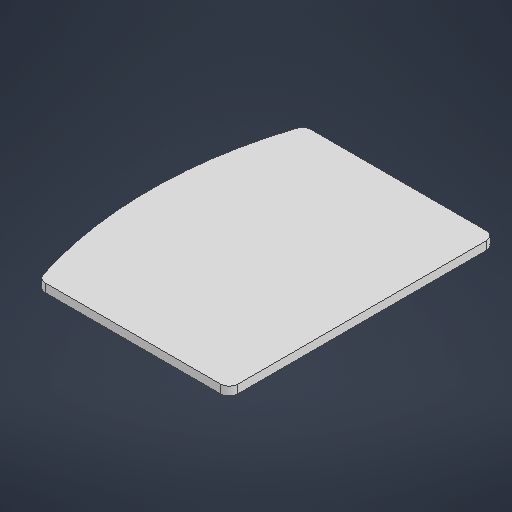
# Autodesk Inventor part: Motorplatine
Saved by Autodesk Inventor 2025.3 (Build 293356000, 356)
## iProperties
Created: 2025-05-31
Part Number: Motorplatine
Material: Generisch
Document SubType Name: Modeling
Designer: theod
Density: 1 g/cm^3
Appearance: Vorgabe
Author: theod
Autodesk Inventor part; units mm, degrees
ref_plane "YZ Plane" through (0, 0, 0) normal (1, 0, 0) x (0, 1, 0)
ref_plane "XZ Plane" through (0, 0, 0) normal (0, 1, 0) x (-1, 0, 0)
ref_plane "XY Plane" through (0, 0, 0) normal (0, 0, 1) x (1, 0, 0)
sketch "Skizze1" plane through (0, 0, 0) normal (0, 0, 1) x (1, 0, 0)
  circle A0 centre (-39, 91.781) radius 1.6
  circle A1 centre (39, 91.781) radius 1.6
  circle A2 centre (-44.3776, -92.6293) radius 1.6
  circle A3 centre (92.6293, 44.3776) radius 1.6
  circle A4 centre (-92.6293, -44.3776) radius 1.6
  circle A5 centre (44.3776, -92.6293) radius 1.6
  circle A6 centre (92.6293, -44.3776) radius 1.6
  circle A7 centre (-92.6293, 44.3776) radius 1.6
  arc A8 (-95.4893, -49.3765) -> (-92.2985, -49.8721) centre (-93.7128, -48.4579) ccw
  line L0 (-90.1561, -47.7297) -> (-92.2985, -49.8721)
  arc A9 (-76.014, -47.7297) -> (-90.1561, -47.7297) centre (-83.085, -54.8008) ccw
  line L1 (-47.7297, -76.014) -> (-76.014, -47.7297)
  arc A10 (-47.7297, -90.1561) -> (-47.7297, -76.014) centre (-54.8008, -83.085) ccw
  line L2 (-49.8721, -92.2985) -> (-47.7297, -90.1561)
  arc A11 (-49.8721, -92.2985) -> (-49.3766, -95.4893) centre (-48.4579, -93.7128) ccw
  arc A12 (-49.3766, -95.4893) -> (49.3765, -95.4893) centre (0, 0) ccw
  arc A13 (49.3765, -95.4893) -> (49.8721, -92.2985) centre (48.4579, -93.7128) ccw
  line L3 (47.7297, -90.1561) -> (49.8721, -92.2985)
  arc A14 (47.7297, -76.014) -> (47.7297, -90.1561) centre (54.8008, -83.085) ccw
  line L4 (76.014, -47.7297) -> (47.7297, -76.014)
  arc A15 (90.1561, -47.7297) -> (76.014, -47.7297) centre (83.085, -54.8008) ccw
  line L5 (92.2985, -49.8721) -> (90.1561, -47.7297)
  arc A16 (92.2985, -49.8721) -> (95.4893, -49.3766) centre (93.7128, -48.4579) ccw
  arc A17 (95.4893, -49.3766) -> (95.4893, 49.3765) centre (0, 0) ccw
  arc A18 (95.4893, 49.3765) -> (92.2985, 49.8721) centre (93.7128, 48.4579) ccw
  line L6 (90.1561, 47.7297) -> (92.2985, 49.8721)
  arc A19 (76.014, 47.7297) -> (90.1561, 47.7297) centre (83.085, 54.8008) ccw
  line L7 (47.7297, 76.014) -> (76.014, 47.7297)
  arc A20 (47.7297, 90.1561) -> (47.7297, 76.014) centre (54.8008, 83.085) ccw
  line L8 (49.8721, 92.2985) -> (47.7297, 90.1561)
  arc A21 (49.8721, 92.2985) -> (49.3766, 95.4893) centre (48.4579, 93.7128) ccw
  arc A22 (49.3766, 95.4893) -> (38.3499, 100.4268) centre (0, 0) ccw
  arc A23 (38.3499, 100.4268) -> (35.7063, 99.0826) centre (37.6364, 98.5584) ccw
  arc A24 (28.7451, 85.4847) -> (35.7063, 99.0826) centre (0, 108.781) ccw
  arc A25 (20.9762, 81.781) -> (28.7451, 85.4847) centre (20.9762, 91.781) ccw
  line L9 (20.9762, 81.781) -> (-20.9762, 81.781)
  arc A26 (-28.7451, 85.4847) -> (-20.9762, 81.781) centre (-20.9762, 91.781) ccw
  arc A27 (-35.7063, 99.0826) -> (-28.7451, 85.4847) centre (0, 108.781) ccw
  arc A28 (-35.7063, 99.0826) -> (-38.3499, 100.4268) centre (-37.6364, 98.5584) ccw
  arc A29 (-38.3499, 100.4268) -> (-49.3765, 95.4893) centre (0, 0) ccw
  arc A30 (-49.3765, 95.4893) -> (-49.8721, 92.2985) centre (-48.4579, 93.7128) ccw
  line L10 (-47.7297, 90.1561) -> (-49.8721, 92.2985)
  arc A31 (-47.7297, 76.014) -> (-47.7297, 90.1561) centre (-54.8008, 83.085) ccw
  line L11 (-76.014, 47.7297) -> (-47.7297, 76.014)
  arc A32 (-90.1561, 47.7297) -> (-76.014, 47.7297) centre (-83.085, 54.8008) ccw
  line L12 (-92.2985, 49.8721) -> (-90.1561, 47.7297)
  arc A33 (-92.2985, 49.8721) -> (-95.4893, 49.3766) centre (-93.7128, 48.4579) ccw
  arc A34 (-95.4893, 49.3766) -> (-95.4893, -49.3765) centre (0, 0) ccw
  circle A35 centre (-67.8822, 48.7904) radius 1.6
  circle A36 centre (-48.7904, 67.8822) radius 1.6
  circle A37 centre (-67.8822, -48.7904) radius 1.6
  circle A38 centre (-48.7904, -67.8823) radius 1.6
  circle A39 centre (48.7904, -67.8823) radius 1.6
  circle A40 centre (67.8823, -48.7904) radius 1.6
  circle A41 centre (67.8823, 48.7904) radius 1.6
  circle A42 centre (48.7904, 67.8822) radius 1.6
  line L13 (48.7904, 67.8822) -> (67.8823, 48.7904) construction
  line L14 (70.7107, 45.9619) -> (45.9619, 70.7107) construction
  line L15 (67.1751, 42.4264) -> (42.4264, 67.1751)
  line L16 (42.4264, 67.1751) -> (49.4975, 74.2462)
  line L17 (49.4975, 74.2462) -> (74.2462, 49.4975)
  line L18 (74.2462, 49.4975) -> (67.1751, 42.4264)
  line L19 (67.1751, 42.4264) -> (49.4975, 74.2462) construction
  line L20 (42.4264, 67.1751) -> (74.2462, 49.4975) construction
  line L21 (0, 0) -> (61.8718, 61.8718) construction
  line L22 (61.8718, 61.8718) -> (13.7886, 13.7886) construction
  line L23 (67.5287, 56.215) -> (19.4454, 8.1317)
  line L24 (19.4454, 8.1317) -> (8.1317, 19.4454)
  line L25 (8.1317, 19.4454) -> (56.215, 67.5287)
  line L26 (56.215, 67.5287) -> (67.5287, 56.215)
  line L27 (67.5287, 56.215) -> (8.1317, 19.4454) construction
  line L28 (19.4454, 8.1317) -> (56.215, 67.5287) construction
  line L29 (-74.2462, 49.4975) -> (-49.4975, 74.2462)
  line L30 (-49.4975, 74.2462) -> (-42.4264, 67.1751)
  line L31 (-56.215, 67.5287) -> (-8.1317, 19.4454)
  line L32 (-42.4264, 67.1751) -> (-67.1751, 42.4264)
  line L33 (-19.4454, 8.1317) -> (-67.5287, 56.215)
  line L34 (-67.1751, 42.4264) -> (-74.2462, 49.4975)
  line L35 (-8.1317, 19.4454) -> (-19.4454, 8.1317)
  line L36 (-49.4975, -74.2462) -> (-74.2462, -49.4975)
  line L37 (-74.2462, -49.4975) -> (-67.1751, -42.4264)
  line L38 (-67.5287, -56.215) -> (-19.4454, -8.1317)
  line L39 (-67.1751, -42.4264) -> (-42.4264, -67.1751)
  line L40 (-8.1317, -19.4454) -> (-56.215, -67.5287)
  line L41 (-42.4264, -67.1751) -> (-49.4975, -74.2462)
  line L42 (-19.4454, -8.1317) -> (-8.1317, -19.4454)
  line L43 (74.2462, -49.4975) -> (49.4975, -74.2462)
  line L44 (49.4975, -74.2462) -> (42.4264, -67.1751)
  line L45 (56.215, -67.5287) -> (8.1317, -19.4454)
  line L46 (42.4264, -67.1751) -> (67.1751, -42.4264)
  line L47 (19.4454, -8.1317) -> (67.5287, -56.215)
  line L48 (67.1751, -42.4264) -> (74.2462, -49.4975)
  line L49 (8.1317, -19.4454) -> (19.4454, -8.1317)
  circle A43 centre (-14.902, -0.6571) radius 1.4
  circle A44 centre (14.732, 5.2251) radius 1.4
  circle A45 centre (0, 0) radius 4.85
  circle A46 centre (-22.9365, 16.8843) radius 1.6
  circle A47 centre (-22.9365, 16.8843) radius 1.6
  circle A48 centre (22.7665, 22.7665) radius 1.6
  circle A49 centre (22.7665, 22.7665) radius 1.6
  circle A50 centre (22.7665, -28.6487) radius 1.6
  circle A51 centre (22.7665, -28.6487) radius 1.6
  circle A52 centre (-22.7665, -22.7665) radius 1.6
  circle A53 centre (-22.7665, -22.7665) radius 1.6
  line L50 (-22.9365, 16.8843) -> (-25.9365, 16.8843)
  line L51 (-25.9365, 16.8843) -> (-25.9365, 19.8843)
  line L52 (-22.9365, 16.8843) -> (-22.9365, 13.8843)
  line L53 (-22.9365, 13.8843) -> (-19.9365, 13.8843)
  line L54 (22.7665, -28.6487) -> (25.7665, -28.6487)
  line L55 (25.7665, -28.6487) -> (25.7665, -31.6487)
  line L56 (22.7665, -28.6487) -> (22.7665, -25.6487)
  line L57 (22.7665, -25.6487) -> (19.7665, -25.6487)
  line L58 (-25.9365, 19.8843) -> (25.7665, 19.8843)
  line L59 (25.7665, 19.8843) -> (25.7665, -31.6487)
  line L60 (25.7665, -31.6487) -> (-25.9365, -31.6487)
  line L61 (-25.9365, -31.6487) -> (-25.9365, 19.8843)
  line L62 (19.7665, -25.6487) -> (-19.9365, -25.6487)
  line L63 (-19.9365, -25.6487) -> (-19.9365, 13.8843)
  line L64 (-19.9365, 13.8843) -> (19.7665, 13.8843)
  line L65 (19.7665, 13.8843) -> (19.7665, -25.6487)
  line L66 (-14.902, -0.6571) -> (-14.902, -2.6571)
  line L67 (-14.902, -2.6571) -> (-14.902, 1.3429)
  line L68 (-14.902, 1.3429) -> (-19.9365, 1.3429)
  line L69 (-14.902, -2.6571) -> (-19.9365, -2.6571)
  circle A54 centre (-14.902, -0.6571) radius 2
  line L70 (0, 4.85) -> (0, 5.85)
  line L71 (14.902, -2.6571) -> (19.9365, -2.6571)
  circle A55 centre (14.902, -0.6571) radius 2
  line L72 (14.902, 1.3429) -> (19.9365, 1.3429)
  circle A56 centre (14.902, -0.6571) radius 1.4
  line L73 (-97.5, 3.1883) -> (-25.9365, -5.8822) construction
  line L74 (-47.1904, -35.8767) -> (-47.1904, 29.5) construction
  line L75 (-107.5, 0) -> (-97.5, 3.1883) construction
  line L76 (-47.1904, -3.1883) -> (-97.5, 3.1883) construction
  line L77 (-90.8295, -31.5) -> (-49.1904, -31.5)
  line L78 (-47.1904, -29.5) -> (-47.1904, 31.5)
  line L79 (-49.1904, 31.5) -> (-90.8295, 31.5)
  line L80 (-93.745, -26.7978) -> (-47.1904, 31.5) construction
  line L81 (-47.1904, -31.5) -> (-93.745, 26.7978) construction
  arc A57 (-92.7317, 30.1178) -> (-92.7317, -30.1178) centre (0, 0) ccw
  arc A58 (-49.1904, -31.5) -> (-47.1904, -29.5) centre (-49.1904, -29.5) ccw
  arc A59 (-47.1904, 29.5) -> (-49.1904, 31.5) centre (-49.1904, 29.5) ccw
  arc A60 (-92.7317, -30.1178) -> (-90.8295, -31.5) centre (-90.8295, -29.5) ccw
  arc A61 (-90.8295, 31.5) -> (-92.7317, 30.1178) centre (-90.8295, 29.5) ccw
  line L82 (-47.1904, 0) -> (-97.5, 0)
  point P0 (0, 0)
  point P1 (0, 0)
  point P2 (0, 0)
  point P3 (58.3363, 58.3363)
  point P4 (37.8302, 37.8302)
  point P5 (-61.8718, 61.8718)
  point P6 (-13.7886, 13.7886)
  point P7 (-61.8718, -61.8718)
  point P8 (-13.7886, -13.7886)
  point P9 (61.8718, -61.8718)
  point P10 (13.7886, -13.7886)
  point P11 (0, 0)
  point P12 (-47.1904, 35.8767)
  point P13 (-72.3452, 0)
  point P14 (-92.2713, 31.5)
  point P15 (-92.2713, -31.5)
  dimension "d4" = 3.2
  dimension "d5" = 3.2
  dimension "d6" = 360
  dimension "d7" = 4
  dimension "d8" = 35
  dimension "d9" = 68
  dimension "d10" = 16
  dimension "d11" = 360
  dimension "d13" = 3
  dimension "d14" = 3
  dimension "d15" = 3
  dimension "d16" = 3
  dimension "d17" = 3
  dimension "d18" = 3
  dimension "d19" = 3
  dimension "d20" = 3
  dimension "d21" = 2
  dimension "d22" = 4
  dimension "d23" = 1
  dimension "d25" = 63
  dimension "d28" = 2
  dimension "d29" = 2
  constraints: 166 end point, 70 point on circle, 59 centre point, 16 point on line, 11 parallel, 10 midpoint, 10 perpendicular, 8 tangent, 7 coincident, 6 horizontal, 6 symmetric about line, 6 vertical, 3 vertical alignment, 2 equal radius, 1 collinear, 93 other
  measures "d4" diameter of A35
  measures "d5" diameter of A36
  measures "d7" distance of L13.end L14.start
  measures "d8" distance of L14.start L14.end
  measures "d9" distance of L21.end L22.end
  measures "d10" distance of L23.end L24.end
  measures "d13" distance of L50.start L50.end
  measures "d14" distance of L50.end L51.end
  measures "d15" distance of L50.start L52.end
  measures "d16" distance of L52.end L53.end
  measures "d17" distance of L54.start L54.end
  measures "d18" distance of L54.end L55.end
  measures "d19" distance of L54.start L56.end
  measures "d20" distance of L56.end L57.end
  measures "d21" distance of L66.start L66.end
  measures "d22" distance of L66.end L67.end
  measures "d23" distance of L70.start L70.end
  measures "d25" distance of L78.end L81.start
  measures "d28" radius of A58
  measures "d29" radius of A60
extrude "Extrusion1" add sketch "Skizze1" along normal blind 2 contours A60 A57 L82 L78 A58 L77 | A57 A61 L79 A59 L78 L82
